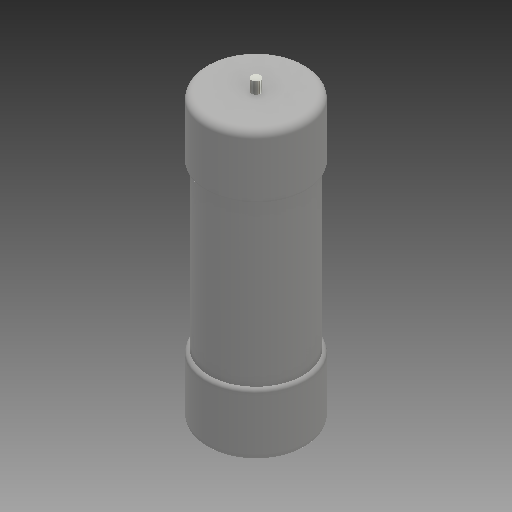
# Autodesk Inventor part: resistor WHS7 68R
Saved by Autodesk Inventor 2017 (Build 210142000, 142)
## iProperties
Part Number: resistor WHS7 68R
Material: Gummi, Silikon
Document SubType Name: Modeling
Designer: ExCISS
Density: 1.25 g/cm^3
Appearance: grau
Mass: 1.93712 g
Surface Area: 9.56822 cm^2
Volume: 1.5497 cm^3
Author: ExCISS
Autodesk Inventor part; units mm, degrees
ref_plane "YZ Plane" through (0, 0, 0) normal (1, 0, 0) x (0, 1, 0)
ref_plane "XZ Plane" through (0, 0, 0) normal (0, 1, 0) x (-1, 0, 0)
ref_plane "XY Plane" through (0, 0, 0) normal (0, 0, 1) x (1, 0, 0)
sketch "Skizze1" plane through (0, 0, 0) normal (0, 0, 1) x (1, 0, 0)
  circle A0 centre (0, 0) radius 4.4
  dimension "d0" = 8.8
  constraints: 1 centre point, 1 coincident
  measures "d0" diameter of A0
extrude "Extrusion1" add sketch "Skizze1" along normal mid plane 25
sketch "Skizze4" plane through (0, 0, 0) normal (0, 0, 1) x (1, 0, 0)
  circle A0 centre (0, 0) radius 4.4 projected
  circle A1 centre (0, 0) radius 4.1
  dimension "d10" = 0.3
  constraints: 1 centre point, 1 coincident
  measures "d10" radial gap between concentric circles of A0 A1
extrude "Extrusion4" cut sketch "Skizze4" along normal mid plane 14
fillet "Rundung1" radius 0.3 2 edges at (-4.4, 0, 7) (-4.4, 0, -7)
fillet "Rundung2" radius 0.6 2 edges at (-4.4, 0, 12.5) (-4.4, 0, -12.5)
sketch "Skizze6" plane through (0, 0, 12.5) normal (0, 0, 1) x (1, 0, 0)
  circle A0 centre (0, 0) radius 0.405
  dimension "d21" = 0.81
  constraints: 1 centre point, 1 coincident
  measures "d21" diameter of A0
extrude "Extrusion6" add sketch "Skizze6" along normal blind 1
mirror "Spiegeln3" about plane through (0, 0, 0) normal (0, 0, 1) of "Extrusion6"
